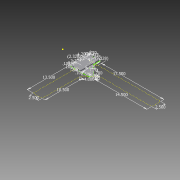
# Autodesk Inventor part: Phone_Holder
Saved by Autodesk Inventor 2013 (Build 170138000, 138)
## iProperties
Created: 2015-03-29
Part Number: Phone_Holder
Material: Generic
Document SubType Name: Modeling
Designer: Pat
Density: 1 g/cm^3
Author: Pat
Autodesk Inventor part; units mm, degrees
ref_plane "YZ Plane" through (0, 0, 0) normal (1, 0, 0) x (0, 1, 0)
ref_plane "XZ Plane" through (0, 0, 0) normal (0, 1, 0) x (-1, 0, 0)
ref_plane "XY Plane" through (0, 0, 0) normal (0, 0, 1) x (1, 0, 0)
sketch "Sketch1" plane through (0, 0, 0) normal (0, 1, 0) x (-1, 0, 0)
  line L0 (-128.4561, -59.0678) -> (-200.4651, -59.0678)
  line L1 (-200.4651, -59.0678) -> (-200.4651, 72.3772)
  line L2 (-200.4651, 72.3772) -> (-128.4561, 72.3772)
  line L3 (-128.4561, 72.3772) -> (-128.4561, 49.0473)
  line L4 (-128.4561, 49.0473) -> (-127.1861, 49.0473)
  line L5 (-127.1861, 49.0473) -> (-127.1861, 38.6333)
  line L6 (-127.1861, 38.6333) -> (-128.4561, 38.6333)
  line L7 (-128.4561, 38.6333) -> (-128.4561, 3.6194)
  line L8 (-128.4561, 3.6194) -> (-127.1861, 3.6194)
  line L9 (-127.1861, 3.6194) -> (-127.1861, -6.7946)
  line L10 (-127.1861, -6.7946) -> (-128.4561, -6.7946)
  line L11 (-128.4561, -6.7946) -> (-128.4561, -20.3074)
  line L12 (-128.4561, -20.3074) -> (-127.1861, -20.3074)
  line L13 (-127.1861, -20.3074) -> (-127.1861, -39.6114)
  line L14 (-127.1861, -39.6114) -> (-128.4561, -39.6114)
  line L15 (-128.4561, -39.6114) -> (-128.4561, -59.0678)
  line L16 (-203.0051, 74.9172) -> (-125.9161, 74.9172)
  line L17 (-125.9161, 74.9172) -> (-125.9161, -61.6078)
  line L18 (-125.9161, -61.6078) -> (-203.0051, -61.6078)
  line L19 (-203.0051, -61.6078) -> (-203.0051, 74.9172)
  circle A0 centre (-164.6511, -28.5878) radius 4.9213 construction
  line L20 (-203.0051, 74.9172) -> (-266.5051, 74.9172)
  line L21 (-164.6511, 373.4543) -> (-228.1511, 373.4543) construction
  line L22 (-228.1511, 373.4543) -> (-228.1511, 106.7543) construction
  line L23 (-228.1511, 106.7543) -> (-299.9932, 34.9122) construction
  line L24 (-299.9932, 34.9122) -> (-668.2932, 34.9122) construction
  line L25 (-668.2932, 34.9122) -> (-668.2932, -28.5878) construction
  line L26 (-668.2932, -28.5878) -> (-223.7932, -28.5878) construction
  line L27 (-223.7932, -28.5878) -> (-164.6511, 30.5543) construction
  line L28 (-164.6511, 30.5543) -> (-164.6511, 373.4543) construction
  line L29 (-264.0722, 70.8332) -> (-194.2222, 0.9832) construction
  line L30 (-164.6511, 30.5543) -> (-164.6511, -28.5878) construction
  line L31 (-164.6511, -28.5878) -> (-223.7932, -28.5878) construction
  circle A1 centre (-251.4998, 58.2609) radius 2.54
  circle A2 centre (-215.5788, 22.3399) radius 1.7653
  line L32 (-266.5051, 74.9172) -> (-266.5051, 49.5172)
  line L33 (-266.5051, 49.5172) -> (-203.0051, -13.9828)
  line L34 (-177.3511, 74.9172) -> (-177.3511, 72.3772)
  line L35 (-151.9511, 74.9172) -> (-151.9511, 72.3772)
  line L36 (-177.3511, -61.6078) -> (-177.3511, -59.0678)
  line L37 (-151.9511, -61.6078) -> (-151.9511, -59.0678)
  line L38 (-266.5051, 68.4003) -> (-259.9882, 74.9172)
  point P0 (0, 0)
  dimension "d0" = 72.009
  dimension "d3" = 131.445
  dimension "d4" = 10.414
  dimension "d5" = 10.414
  dimension "d6" = 19.304
  dimension "d7" = 23.3299
  dimension "d8" = 35.0139
  dimension "d9" = 13.5128
  dimension "d10" = 1.27
  dimension "d11" = 2.54
  dimension "d12" = 2.54
  dimension "d13" = 2.54
  dimension "d14" = 2.54
  dimension "d15" = 9.8425
  dimension "d17" = 36.195
  dimension "d18" = 30.48
  dimension "d19" = 63.5
  dimension "d20" = 63.5
  dimension "d21" = 63.5
  dimension "d22" = 101.6
  dimension "d23" = 266.7
  dimension "d24" = 368.3
  dimension "d25" = 444.5
  dimension "d26" = 342.9
  dimension "d27" = 5.08
  dimension "d28" = 3.5306
  dimension "d29" = 17.78
  dimension "d30" = 68.58
  dimension "d31" = 25.4
  dimension "d44" = 12.7
  dimension "d45" = 12.7
  dimension "d64" = 59.142
  dimension "d65" = 59.142
  constraints: 78 end point, 22 parallel, 15 point on line, 11 perpendicular, 6 collinear, 3 centre point, 2 horizontal, 2 midpoint, 1 coincident
  measures "d0" distance of L0.start L0.end
  measures "d3" distance of L0.end L1.end
  measures "d4" distance of L4.end L5.end
  measures "d5" distance of L8.end L9.end
  measures "d6" distance of L12.end L13.end
  measures "d7" distance of L2.end L3.end
  measures "d8" distance of L6.end L7.end
  measures "d9" distance of L10.end L11.end
  measures "d10" distance of L13.end L14.end
  measures "d11" horizontal distance of L16.end L2.end
  measures "d12" horizontal distance of L1.end L16.start
  measures "d13" horizontal distance of L2.end L16.end
  measures "d14" horizontal distance of L17.end L0.start
  measures "d15" diameter of A0
  measures "d17" horizontal distance of A0.centre L0.start
  measures "d18" vertical distance of L0.start A0.centre
  measures "d19" distance of L16.start L20.end
  measures "d20" distance of L21.start L21.end
  measures "d21" distance of L24.end L25.end
  measures "d22" distance of L22.end L23.end
  measures "d23" distance of L21.end L22.end
  measures "d24" distance of L23.end L24.end
  measures "d25" distance of L25.end L26.end
  measures "d26" distance of L27.end L21.start
  measures "d27" diameter of A1
  measures "d28" diameter of A2
  measures "d29" distance from line of L23 A1.centre
  measures "d30" distance from line of L23 A2.centre
  measures "d31" distance of L20.end L32.end
  measures "d44" distance between parallel lines of L28 L34
  measures "d45" distance between parallel lines of L28 L35
  measures "d64" distance of A0.centre L26.end
  measures "d65" distance of L27.end L30.end
extrude "Extrusion13" add sketch "Sketch1" along normal blind 2.54 contours L0 L1 L2 L3 L4 L5 L6 L7 L8 L9 L10 L11 L12 L13 L14 L15
extrude "Extrusion14" add sketch "Sketch1" along normal blind 3.81 contours L33 L32 L38 L20 L19
extrude "Extrusion15" add sketch "Sketch1" along normal blind 10.16 contours L15 L14 L13 L12 L11 L10 L9 L8 L7 L6 L5 L4 L3 L2 L35 L16 L17 L18 L37 L0 | L36 L18 L19 L16 L34 L2 L1 L0
body "Solid5"
